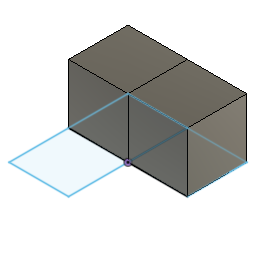
BooleanAdjacent (Autodesk Fusion 360 design; units mm, degrees)
Autodesk Fusion 360 part; units mm, degrees
sketch "Sketch1" plane through (0, 0, 0) normal (0, 0, 1) x (1, 0, 0)
  line L0 (0, 0) -> (-10, 0)
  line L1 (-10, 0) -> (-10, 10)
  line L2 (-10, 10) -> (0, 10)
  line L3 (0, 10) -> (0, 0)
  line L4 (0, 0) -> (10, 0)
  line L5 (10, 0) -> (10, 10)
  line L6 (10, 10) -> (0, 10)
  line L7 (0, 10) -> (0, 0)
  line L8 (-10, 10) -> (0, 10)
  line L9 (0, 10) -> (0, -10)
  line L10 (0, -10) -> (-10, -10)
  line L11 (-10, -10) -> (-10, 10)
  constraint horizontal L0
  constraint vertical L1
  constraint horizontal L2
  constraint vertical L3
  constraint coincident L0.start L3.end
  constraint horizontal L4
  constraint vertical L5
  constraint horizontal L6
  constraint vertical L7
  constraint horizontal L8
  constraint vertical L9
  constraint horizontal L10
  constraint vertical L11
extrude "Extrude1" add sketch "Sketch1" along normal blind 10 contours L3 L4 L5 L6 L7 L9 makes body 1
extrude "Extrude2" add sketch "Sketch1" along normal blind 10 separate body contours L0 L1 L2 L3 L7 L8 L9 L11 makes body 2
